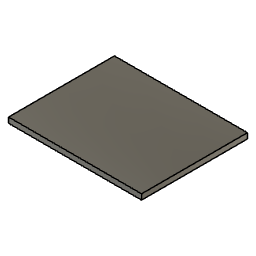
rest_casing_lid v2 (Autodesk Fusion 360 design; units mm, degrees)
Autodesk Fusion 360 part; units mm, degrees
sketch "Sketch1" plane through (0, -4.2959, 0) normal (0, -1, 0) x (1, 0, 0)
  line L0 (-20, 21.5) -> (-25, 21.5)
  line L1 (-25, 21.5) -> (-25, 24)
  line L2 (-25, 24) -> (-20, 24)
  line L3 (-20, 24) -> (-20, 26)
  line L4 (-20, 26) -> (-32, 26)
  line L5 (-32, 26) -> (-32, -1)
  line L6 (-32, -1) -> (32, -1)
  line L7 (32, -1) -> (32, 26)
  line L8 (32, 26) -> (20, 26)
  line L9 (20, 26) -> (20, 24)
  line L10 (20, 24) -> (25, 24)
  line L11 (25, 24) -> (25, 21.5)
  line L12 (25, 21.5) -> (20, 21.5)
  line L13 (20, 21.5) -> (20, 0)
  line L14 (20, 0) -> (-20, 0)
  line L15 (-20, 0) -> (-20, 21.5)
  line L16 (24.5, 21.75) -> (-24.5, 21.75)
  line L17 (-24.5, 21.75) -> (-24.5, 23.75)
  line L18 (-24.5, 23.75) -> (24.5, 23.75)
  line L19 (24.5, 23.75) -> (24.5, 21.75)
  line L20 (24.5, 21.75) -> (-24.5, 23.75) construction
  line L21 (-24.5, 21.75) -> (24.5, 23.75) construction
  point P0 (0, 22.75)
  dimension "d64" = 49
  dimension "d65" = 2
  dimension "d66" = 2.25
  dimension "d67" = 0.5
  constraint horizontal L16
  constraint perpendicular L16 L17
  constraint parallel L16 L18
  constraint parallel L17 L19
  constraint coincident L20 P0
  constraint coincident L21 P0
  measures "d64" distance of L17.end L18.end
  measures "d65" distance of L16.end L17.end
  measures "d66" distance of L8 L18
  measures "d67" distance of L11 L19
extrude "Extrude1" add sketch "Sketch1" against normal blind 39 contours L16 L17 L18 L19
